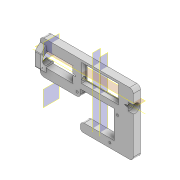
# Autodesk Inventor part: 10_Wellplate_base_v2
Saved by Autodesk Inventor 2022 (Build 260153000, 153)
## iProperties
Created: 2022-04-18
Part Number: 10_Wellplate_base_v2
Material: Generic
Document SubType Name: Modeling
Designer: Prakash Lab
Density: 1 g/cm^3
Appearance: Default
Author: Prakash Lab
Autodesk Inventor part; units mm, degrees
ref_plane "YZ Plane" through (0, 0, 0) normal (1, 0, 0) x (0, 1, 0)
ref_plane "XZ Plane" through (0, 0, 0) normal (0, 1, 0) x (-1, 0, 0)
ref_plane "XY Plane" through (0, 0, 0) normal (0, 0, 1) x (1, 0, 0)
sketch "Sketch1" plane through (0, 0, 0) normal (0, 0, 1) x (1, 0, 0)
  line L0 (63.9, -42.75) -> (-63.9, -42.75)
  line L1 (-63.9, -42.75) -> (-63.9, 42.75)
  line L2 (-63.9, 42.75) -> (63.9, 42.75)
  line L3 (63.9, 42.75) -> (63.9, -42.75)
  line L4 (63.9, -42.75) -> (-63.9, 42.75) construction
  line L5 (-63.9, -42.75) -> (63.9, 42.75) construction
  point P0 (0, 0)
  dimension "d0" = 127.8
  dimension "d1" = 85.5
  constraints: 12 end point, 2 midpoint, 2 parallel, 1 horizontal, 1 perpendicular
  measures "d0" distance of L0.start L0.end
  measures "d1" distance of L0.end L1.end
extrude "Extrusion1" add sketch "Sketch1" along normal blind 10
fillet "Fillet1" radius 4 4 edges at (63.9, 42.75, 5) (-63.9, 42.75, 5) (-63.9, -42.75, 5) (63.9, -42.75, 5)
sketch "Sketch2" plane through (0, 0, 10) normal (0, 0, 1) x (1, 0, 0)
  arc A0 (59.9, -42.75) -> (63.9, -38.75) centre (59.9, -38.75) ccw projected
  line L0 (63.9, -38.75) -> (63.9, 38.75) projected
  arc A1 (63.9, 38.75) -> (59.9, 42.75) centre (59.9, 38.75) ccw projected
  line L1 (59.9, 42.75) -> (-59.9, 42.75) projected
  arc A2 (-59.9, 42.75) -> (-63.9, 38.75) centre (-59.9, 38.75) ccw projected
  line L2 (-63.9, 38.75) -> (-63.9, -38.75) projected
  arc A3 (-63.9, -38.75) -> (-59.9, -42.75) centre (-59.9, -38.75) ccw projected
  line L3 (-59.9, -42.75) -> (59.9, -42.75) projected
  line L4 (43.9, 4.75) -> (-7.1, 4.75)
  line L5 (-7.1, 4.75) -> (-7.1, 29.75)
  line L6 (-7.1, 29.75) -> (43.9, 29.75)
  line L7 (43.9, 29.75) -> (43.9, 4.75)
  line L8 (43.9, 4.75) -> (-7.1, 29.75) construction
  line L9 (-7.1, 4.75) -> (43.9, 29.75) construction
  point P0 (0, 0)
  point P1 (18.4, 17.25)
  dimension "d5" = 51
  dimension "d6" = 25
  dimension "d7" = 20
  dimension "d8" = 13
  constraints: 12 end point, 2 midpoint, 2 parallel, 1 horizontal, 1 perpendicular
  measures "d5" distance of L5.end L6.end
  measures "d6" distance of L4.end L5.end
  measures "d7" distance between parallel lines of L0 L7
  measures "d8" distance between parallel lines of L6 L1
extrude "Extrusion2" cut sketch "Sketch2" against normal blind 6 contours L4 L5 L6 L7
sketch "Sketch3" plane through (0, 0, 4) normal (0, 0, 1) x (1, 0, 0)
  line L0 (-7.1, 29.75) -> (43.9, 29.75) projected
  line L1 (-7.1, 4.75) -> (-7.1, 29.75) projected
  line L2 (43.9, 4.75) -> (-7.1, 4.75) projected
  line L3 (43.9, 29.75) -> (43.9, 4.75) projected
  line L4 (42.4, 28.25) -> (-5.6, 28.25)
  line L5 (-5.6, 28.25) -> (-5.6, 6.25)
  line L6 (-5.6, 6.25) -> (42.4, 6.25)
  line L7 (42.4, 6.25) -> (42.4, 28.25)
  point P0 (0, 0)
  dimension "d11" = 1.5
  constraints: 8 end point, 3 other
  measures "d11" distance between parallel lines of L0 L4
extrude "Extrusion3" cut sketch "Sketch3" against normal through all contours L7 L6 L5 L4
ref_plane "Work Plane1" through (18.4, 4.75, 10) normal (-1, 0, 0) x (0, 0, 1)
ref_plane "Work Plane2" through (-7.1, 17.25, 10) normal (0, 1, 0) x (1, 0, 0)
chamfer "Chamfer1" distance 4 angle 45 4 edges at (18.4, 6.25, 0) (42.4, 17.25, 0) (18.4, 28.25, 0) (-5.6, 17.25, 0)
ref_plane "Work Plane3" through (8.4, 4.75, 10) normal (-1, 0, 0) x (0, 0, 1)
sketch "Sketch12" plane through (63.9, -38.75, 0) normal (1, 0, 0) x (0, 0, -1)
  circle A0 centre (-7.125, 48) radius 4.2 construction
  circle A1 centre (-7.125, 48) radius 3.5
  point P0 (0, 38.75)
  dimension "d100" = 7
  constraints: 1 centre point
  measures "d100" diameter of A1
extrude "Extrusion12" cut sketch "Sketch12" against normal blind 30 draft -3
sketch "Sketch13" plane through (63.9, -38.75, 0) normal (1, 0, 0) x (0, 0, -1)
  arc A0 (-10, 44.9382) -> (-10, 51.0618) centre (-7.125, 48) ccw projected
  circle A1 centre (-7.125, 48) radius 6
  point P0 (0, 38.75)
  dimension "d63" = 12
  constraints: 1 centre point, 1 coincident
  measures "d63" diameter of A1
extrude "Extrusion13" cut sketch "Sketch13" against normal blind 7
mirror "Mirror1" about plane through (18.4, 4.75, 10) normal (-1, 0, 0) of "Extrusion12", "Extrusion13"
ref_plane "Work Plane4" through (-47.9, 27.75, 11) normal (-1, 0, 0) x (0, 0, 1)
ref_plane "Work Plane5" through (-39.7, 19.25, 21) normal (0, 0, 1) x (1, 0, 0)
ref_plane "Arbeitsebene7" through (-58.9, -38.75, 0) normal (-1, 0, 0) x (0, 0, 1)
sketch "Skizze28" plane through (-58.9, -38.75, 0) normal (-1, 0, 0) x (0, 0, 1)
  line L0 (17.125, 56.5) -> (17.125, 39.5) projected
  arc A0 (17.125, 56.5) -> (15.625, 58) centre (15.625, 56.5) ccw projected
  line L1 (-1.375, 58) -> (15.625, 58) projected
  arc A1 (-1.375, 58) -> (-2.875, 56.5) centre (-1.375, 56.5) ccw projected
  line L2 (-2.875, 39.5) -> (-2.875, 56.5) projected
  arc A2 (-2.875, 39.5) -> (-1.375, 38) centre (-1.375, 39.5) ccw projected
  line L3 (15.625, 38) -> (-1.375, 38) projected
  arc A3 (15.625, 38) -> (17.125, 39.5) centre (15.625, 39.5) ccw projected
  circle A4 centre (15.125, 56) radius 0.7835 projected
  circle A5 centre (15.125, 40) radius 0.7835 projected
  circle A6 centre (-0.875, 56) radius 0.7835 projected
  circle A7 centre (-0.875, 40) radius 0.7835 projected
  circle A8 centre (7.125, 48) radius 7.5 projected
  arc A9 (17.625, 56.5) -> (15.625, 58.5) centre (15.625, 56.5) ccw
  line L4 (17.625, 56.5) -> (17.625, 39.5)
  arc A10 (15.625, 37.5) -> (17.625, 39.5) centre (15.625, 39.5) ccw
  line L5 (15.625, 37.5) -> (-1.375, 37.5)
  arc A11 (-3.375, 39.5) -> (-1.375, 37.5) centre (-1.375, 39.5) ccw
  line L6 (-3.375, 39.5) -> (-3.375, 56.5)
  arc A12 (-1.375, 58.5) -> (-3.375, 56.5) centre (-1.375, 56.5) ccw
  line L7 (-1.375, 58.5) -> (15.625, 58.5)
  point P0 (0, 38.75)
  dimension "d142" = 0.5
  constraints: 8 end point, 8 point on circle, 4 centre point, 7 other
  measures "d142" distance between parallel lines of L1 L7
extrude "Extrusion27" cut sketch "Skizze28" against normal blind 40 contours L0 A3 L3 A2 L2 A1 L1 A0 | A4 | A5 | A6 | A7 | A8 | L4 A10 L5 A11 L6 A12 L7 A9
sketch "Skizze29" plane through (-63.9, -38.75, 0) normal (-1, 0, 0) x (0, 0, 1)
  line L0 (17.125, 56.5) -> (17.125, 39.5) projected
  arc A0 (17.125, 56.5) -> (15.625, 58) centre (15.625, 56.5) ccw projected
  line L1 (-1.375, 58) -> (15.625, 58) projected
  arc A1 (-1.375, 58) -> (-2.875, 56.5) centre (-1.375, 56.5) ccw projected
  line L2 (-2.875, 39.5) -> (-2.875, 56.5) projected
  arc A2 (-2.875, 39.5) -> (-1.375, 38) centre (-1.375, 39.5) ccw projected
  line L3 (15.625, 38) -> (-1.375, 38) projected
  arc A3 (15.625, 38) -> (17.125, 39.5) centre (15.625, 39.5) ccw projected
  circle A4 centre (15.125, 56) radius 0.7835 projected
  circle A5 centre (15.125, 40) radius 0.7835 projected
  circle A6 centre (-0.875, 56) radius 0.7835 projected
  circle A7 centre (-0.875, 40) radius 0.7835 projected
  circle A8 centre (7.125, 48) radius 7.5 projected
  line L4 (0, 77.5) -> (0, 0) projected
  line L5 (10, 77.5) -> (10, 0) projected
  line L6 (10, 0) -> (10, 42.7337) projected
  line L7 (10, 31.7537) -> (16.6857, 38.4393)
  line L8 (16.6857, 57.5607) -> (10, 64.2463)
  line L9 (10, 68.5) -> (10, 31.5) projected
  point P0 (0, 38.75)
  point P1 (0, 58)
  point P2 (0, 38)
  point P3 (10, 11.9077)
  point P4 (10, 38)
  point P5 (10, 58)
  point P6 (10, 10.3787)
  dimension "d151" = 45
  dimension "d152" = 45
  constraints: 4 end point, 2 point on circle, 2 point on line
  measures "d151" angle of L1 L8
  measures "d152" angle of L3 L7
extrude "Extrusion28" add sketch "Skizze29" against normal blind 8 contours L0 A3 L3 L5 A8 L1 A0 | A0 L1 L5 L8 | L7 L5 L3 A3 | L5 A8 L4 L1 | L3 L4 A8 L5 | L5 A8 L4 | A8 L5
sketch "Skizze30" plane through (-55.9, -38.75, 0) normal (1, 0, 0) x (0, 0, -1)
  circle A0 centre (-7.125, 48) radius 7.3 projected
  circle A1 centre (-7.125, 48) radius 7.8
  point P0 (0, 38.75)
  dimension "d147" = 0.5
  constraints: 1 centre point
  measures "d147" radial gap between concentric circles of A0 A1
extrude "Extrusion29" cut sketch "Skizze30" against normal up to surface (8 mm away) contours A0 | A1
fillet "Rundung6" radius 2 2 edges at (-59.9, 6.076, 0) (-59.9, 12.424, 0)
sketch "Skizze40" plane through (0, 0, 10) normal (0, 0, 1) x (1, 0, 0)
  line L0 (-55.9, -1.25) -> (-55.9, -6.9963) projected
  line L1 (-55.9, -6.9963) -> (-63.9, -6.9963) projected
  line L2 (-63.9, -6.9963) -> (-63.9, -38.75) projected
  arc A0 (-63.9, -38.75) -> (-59.9, -42.75) centre (-59.9, -38.75) ccw projected
  line L3 (-59.9, -42.75) -> (59.9, -42.75) projected
  arc A1 (59.9, -42.75) -> (63.9, -38.75) centre (59.9, -38.75) ccw projected
  line L4 (63.9, -38.75) -> (63.9, 3.9837) projected
  line L5 (63.9, 3.9837) -> (56.9, 3.9837) projected
  line L6 (56.9, 3.9837) -> (56.9, 8.0046) projected
  line L7 (56.9, 10.4954) -> (56.9, 14.5163) projected
  line L8 (56.9, 14.5163) -> (63.9, 14.5163) projected
  line L9 (63.9, 14.5163) -> (63.9, 38.75) projected
  arc A2 (63.9, 38.75) -> (59.9, 42.75) centre (59.9, 38.75) ccw projected
  line L10 (59.9, 42.75) -> (-59.9, 42.75) projected
  arc A3 (-59.9, 42.75) -> (-63.9, 38.75) centre (-59.9, 38.75) ccw projected
  line L11 (-63.9, 38.75) -> (-63.9, 25.4963) projected
  line L12 (-63.9, 25.4963) -> (-55.9, 25.4963) projected
  line L13 (-55.9, 25.4963) -> (-55.9, 19.75) projected
  line L14 (-55.9, 19.75) -> (-18.9, 19.75) projected
  line L15 (-18.9, 19.75) -> (-18.9, 10.3274) projected
  line L16 (-18.9, 8.1726) -> (-18.9, -1.25) projected
  line L17 (-18.9, -1.25) -> (-55.9, -1.25) projected
  line L18 (63.9, 14.5163) -> (63.9, 38.75) projected
  line L19 (-63.9, 42.75) -> (63.9, 42.75)
  line L20 (63.9, 42.75) -> (63.9, 32.75)
  line L21 (63.9, 32.75) -> (-63.9, 32.75)
  line L22 (-63.9, 32.75) -> (-63.9, 42.75)
  point P0 (0, 0)
  point P1 (-59.9, 42.75)
  dimension "d178" = 10
  constraints: 8 end point, 2 parallel, 2 vertical alignment, 1 horizontal, 1 perpendicular, 1 point on line
  measures "d178" distance of L19.end L20.end
extrude "Extrusion37" cut sketch "Skizze40" against normal through all
sketch "Skizze41" plane through (0, 0, 10) normal (0, 0, 1) x (1, 0, 0)
  line L0 (63.9, 32.75) -> (-63.9, 32.75) projected
  line L1 (-63.9, 32.75) -> (-63.9, 25.4963) projected
  line L2 (-63.9, 25.4963) -> (-55.9, 25.4963) projected
  line L3 (-55.9, 25.4963) -> (-55.9, 19.75) projected
  line L4 (-55.9, 19.75) -> (-18.9, 19.75) projected
  line L5 (-18.9, 19.75) -> (-18.9, 10.3274) projected
  line L6 (-18.9, 8.1726) -> (-18.9, -1.25) projected
  line L7 (-18.9, -1.25) -> (-55.9, -1.25) projected
  line L8 (-55.9, -1.25) -> (-55.9, -6.9963) projected
  line L9 (-55.9, -6.9963) -> (-63.9, -6.9963) projected
  line L10 (-63.9, -6.9963) -> (-63.9, -38.75) projected
  arc A0 (-63.9, -38.75) -> (-59.9, -42.75) centre (-59.9, -38.75) ccw projected
  line L11 (-59.9, -42.75) -> (59.9, -42.75) projected
  arc A1 (59.9, -42.75) -> (63.9, -38.75) centre (59.9, -38.75) ccw projected
  line L12 (63.9, -38.75) -> (63.9, 3.9837) projected
  line L13 (63.9, 3.9837) -> (56.9, 3.9837) projected
  line L14 (56.9, 3.9837) -> (56.9, 8.0046) projected
  line L15 (56.9, 10.4954) -> (56.9, 14.5163) projected
  line L16 (56.9, 14.5163) -> (63.9, 14.5163) projected
  line L17 (63.9, 14.5163) -> (63.9, 32.75) projected
  line L18 (-63.9, -38.75) -> (63.9, -38.75)
  line L19 (63.9, -38.75) -> (63.9, -52.75)
  line L20 (63.9, -52.75) -> (-63.9, -52.75)
  line L21 (-63.9, -52.75) -> (-63.9, -38.75)
  point P0 (0, 0)
  dimension "d181" = 14
  constraints: 8 end point, 2 parallel, 2 vertical alignment, 1 horizontal, 1 perpendicular
  measures "d181" distance of L18.end L19.end
extrude "Extrusion38" add sketch "Skizze41" against normal up to surface (10 mm away) contours A0 L11 A1 L19 L20 L21
fillet "Rundung7" radius 5 4 edges at (-63.9, 32.75, 5) (63.9, 32.75, 5) (-63.9, -52.75, 5) (63.9, -52.75, 5)
sketch "Skizze42" plane through (0, 0, 10) normal (0, 0, 1) x (1, 0, 0)
  line L0 (34.4, -35.4236) -> (34.4, -18.1764)
  arc A0 (30.4, -35.4236) -> (34.4, -35.4236) centre (32.4, -35.4236) ccw
  line L1 (30.4, -18.1764) -> (30.4, -35.4236)
  arc A1 (34.4, -18.1764) -> (30.4, -18.1764) centre (32.4, -18.1764) ccw
  line L2 (25.4, -35.4236) -> (25.4, -23.25)
  arc A2 (25.4, -35.4236) -> (25.7804, -37.6997) centre (32.4, -35.4236) ccw
  arc A3 (23.8891, -40.35) -> (25.7804, -37.6997) centre (23.8891, -38.35) ccw
  line L3 (37.373, -40.35) -> (23.8891, -40.35)
  arc A4 (37.373, -40.35) -> (37.4, -40.3226) centre (32.4, -35.4236) ccw
  line L4 (37.4, -13.2774) -> (37.4, -40.3226)
  arc A5 (37.4, -13.2774) -> (37.373, -13.25) centre (32.4, -18.1764) ccw
  line L5 (27.427, -13.25) -> (37.373, -13.25)
  arc A6 (27.427, -13.25) -> (27.4, -13.2774) centre (32.4, -18.1764) ccw
  line L6 (27.4, -21.25) -> (27.4, -13.2774)
  arc A7 (25.4, -23.25) -> (27.4, -21.25) centre (25.4, -21.25) ccw
  arc A8 (12.0825, -23.5243) -> (11.6348, -23.331) centre (11.0716, -25.25) ccw
  spline S0 degree 3 poles (12.0825, -23.5243) (11.8555, -23.3913) (11.6488, -23.229) (11.2907, -22.8371) (11.1452, -22.6102) (10.9547, -22.1287) (10.906, -21.8824) (10.906, -21.633) knots 0 0 0 0 0.335568 0.335568 0.679419 0.679419 1 1 1 1
  line L7 (10.906, -13.25) -> (10.906, -21.633)
  line L8 (-7.9188, -13.25) -> (10.906, -13.25)
  arc A9 (-7.9188, -13.25) -> (-8.1, -13.4342) centre (-3.0199, -18.25) ccw
  line L9 (-8.1, -23.0658) -> (-8.1, -13.4342)
  arc A10 (-8.1, -23.0658) -> (-3.0199, -25.25) centre (-3.0199, -18.25) ccw
  line L10 (6.8199, -25.25) -> (-3.0199, -25.25)
  arc A11 (6.8199, -25.25) -> (11.6348, -23.331) centre (6.8199, -18.25) ccw
  arc A12 (-3.0199, -16.25) -> (-3.0199, -20.25) centre (-3.0199, -18.25) ccw
  line L11 (6.8199, -16.25) -> (-3.0199, -16.25)
  arc A13 (6.8199, -20.25) -> (6.8199, -16.25) centre (6.8199, -18.25) ccw
  line L12 (-3.0199, -20.25) -> (6.8199, -20.25)
  line L13 (11.7188, -23.25) -> (25.4, -23.25)
  arc A14 (6.8199, -25.25) -> (11.7188, -23.25) centre (6.8199, -18.25) ccw
  line L14 (6.8199, -25.25) -> (-3.0199, -25.25)
  arc A15 (-8.1, -23.0658) -> (-3.0199, -25.25) centre (-3.0199, -18.25) ccw
  line L15 (-8.1, -40.35) -> (-8.1, -23.0658)
  line L16 (2.9, -40.35) -> (-8.1, -40.35)
  line L17 (2.9, -34.85) -> (2.9, -40.35)
  line L18 (22.3, -34.85) -> (2.9, -34.85)
  line L19 (22.3, -34.85) -> (22.3, -40.35)
  line L20 (22.3, -40.35) -> (23.8891, -40.35)
  arc A16 (23.8891, -40.35) -> (25.7804, -37.6997) centre (23.8891, -38.35) ccw
  arc A17 (25.4, -35.4236) -> (25.7804, -37.6997) centre (32.4, -35.4236) ccw
  line L21 (25.4, -35.4236) -> (25.4, -23.25)
  line L22 (-8.1, -40.35) -> (37.373, -40.35)
  line L23 (37.373, -40.35) -> (37.373, -13.25)
  line L24 (37.373, -13.25) -> (-8.1, -13.25)
  line L25 (-8.1, -13.25) -> (-8.1, -40.35)
  line L26 (37.873, -40.85) -> (-8.6, -40.85)
  line L27 (-8.6, -40.85) -> (-8.6, -12.75)
  line L28 (-8.6, -12.75) -> (37.873, -12.75)
  line L29 (37.873, -12.75) -> (37.873, -40.85)
  circle A18 centre (6.8199, -8.25) radius 3.25
  circle A19 centre (32.4, -8.25) radius 3.25
  circle A20 centre (-3.0199, -8.25) radius 3.25
  line L30 (-18.1, -3.25) -> (47.4, -3.25)
  line L31 (-8.6, -13.75) -> (37.9, -13.75)
  line L32 (37.9, -13.75) -> (37.9, -2.75)
  line L33 (37.9, -2.75) -> (-8.6, -2.75)
  line L34 (-8.6, -2.75) -> (-8.6, -13.75)
  arc A21 (-63.9, -47.75) -> (-58.9, -52.75) centre (-58.9, -47.75) ccw
  line L35 (-8.6, -13.75) -> (-63.9, -13.75)
  line L36 (-63.9, -13.75) -> (-63.9, -52.75)
  line L37 (-63.9, -52.75) -> (-8.6, -52.75)
  line L38 (-8.6, -52.75) -> (-8.6, -13.75)
  line L39 (-58.9, -52.75) -> (58.9, -52.75)
  line L40 (58.9, -52.75) -> (-58.9, -52.75)
  arc A22 (-8.6, -49.2145) -> (-5.0645, -52.75) centre (-5.0645, -49.2145) ccw
  line L41 (-5.0645, -52.75) -> (-8.6, -49.2145) construction
  line L42 (-5.0645, -52.75) -> (-0.0645, -52.75) construction
  circle A23 centre (42.4, -8.25) radius 3.25
  circle A24 centre (-13.1, -8.25) radius 3.25
  circle A25 centre (31.9736, -46.25) radius 3.25
  line L43 (-18.1, -13.25) -> (27.427, -13.25)
  arc A26 (27.427, -13.25) -> (27.4, -13.2774) centre (32.4, -18.1764) ccw
  line L44 (27.4, -13.2774) -> (27.4, -51.25)
  line L45 (27.4, -51.25) -> (37.4, -51.25)
  line L46 (37.4, -51.25) -> (37.4, -13.2774)
  arc A27 (37.4, -13.2774) -> (37.373, -13.25) centre (32.4, -18.1764) ccw
  line L47 (37.373, -13.25) -> (47.4, -13.25)
  line L48 (47.4, -13.25) -> (47.4, -3.25)
  line L49 (-18.1, -3.25) -> (-18.1, -13.25)
  circle A28 centre (32.4, -35.4236) radius 3.25
  circle A29 centre (32.4, -18.1764) radius 3.25
  point P0 (0, 0)
  point P1 (37.4, -13.25)
  point P2 (37.873, -13.75)
  point P3 (-8.6, -40.85)
  point P4 (-5.0645, -52.75)
  dimension "d185" = 0.5
  dimension "d189" = 5
  dimension "d190" = 135
  constraints: 36 end point, 6 parallel, 3 horizontal, 3 perpendicular, 2 point on circle, 2 point on line, 1 centre point, 1 equal length, 1 tangent, 3 other
  measures "d185" distance between parallel lines of L22 L26
  measures "d189" distance of L41.start L41.end
  measures "d190" angle of L42 L41
extrude "Extrusion39" cut sketch "Skizze42" against normal through all contours A0 L1 A28 L0 | L0 A28 L1 A0 | A28 L1 A29 L0 | A29 L1 A1 L0 | L0 A1 L1 A29 | A2 A3 L20 L19 L18 L17 L16 L15 A10 L10 A11 A8 S0 A14 L13 L2 | L2 A7 L44 L3 A3 A2 | L13 A14 S0 L7 L31 L6 A7 | L6 L31 L23 L3 L44 | L3 L44 L26 L27 L31 L9 L15 L16 L22 L20 | L31 L7 L24 A6 L6 | L6 A6 L5 L23 L31 | L3 A4 L46 L26 L44 | A14 A11 L10 A10 L9 L31 L7 S0 | S0 A8 A14 | L22 L17 L18 L19 | L31 L9 A9 L8 L7 | L31 L4 A4 L23 | L23 A5 L4 L31 | L24 L8 L43 L27 L28 L29 L47 L5 | L31 L27 L43 L25 L9 | L47 L29 L31 L4 A5 | L31 L29 L26 L46 L4 | L38 L37 A21 L36 L35 L27 | A9 L25 L24 | L47 L32 L31 L29 | L29 L28 L34 L30 L32 L47 | A22 L39 L38 | L30 L34 L33 L32 | L11 A13 L12 A12 | A18 | A19 | A20
fillet "Rundung8" radius 5 3 edges at (-63.9, -13.75, 5) (-8.6, -13.75, 5) (-8.6, -40.85, 5)
sketch "Skizze43" plane through (0, 0, 10) normal (0, 0, 1) x (1, 0, 0)
  circle A0 centre (-13.1, -8.25) radius 1.45 projected
  circle A1 centre (42.4, -8.25) radius 1.45 projected
  circle A2 centre (31.9736, -46.25) radius 1.45 projected
  point P0 (0, 0)
extrude "Extrusion40" cut sketch "Skizze43" against normal through all
body "Solid1"
